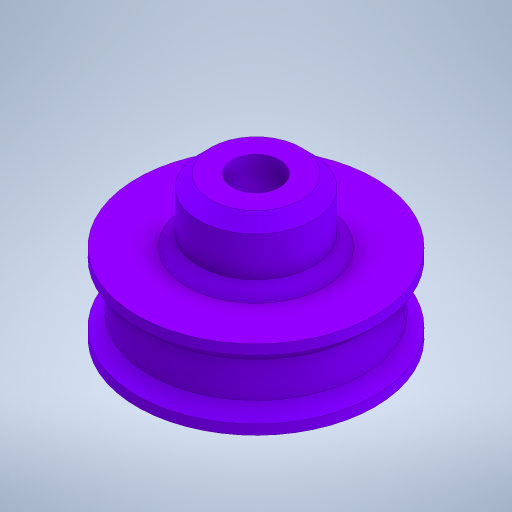
# Autodesk Inventor part: Z Axis Handle
Saved by Autodesk Inventor 2023.1 (Build 271208000, 208)
## iProperties
Created: 2021-10-26
Part Number: Z Axis Handle
Material: Generic
Document SubType Name: Modeling
Designer: xSibe
Density: 1 g/cm^3
Appearance: Plastic Purple
Author: xSibe
Autodesk Inventor part; units mm, degrees
ref_plane "YZ Plane" through (0, 0, 0) normal (1, 0, 0) x (0, 1, 0)
ref_plane "XY Plane" through (0, 0, 0) normal (0, 0, 1) x (1, 0, 0)
sketch "Sketch1" plane through (0, 0, 0) normal (0, 1, 0) x (-1, 0, 0)
  line L0 (1.25, 1.25) -> (-1.25, 1.25)
  line L1 (-1.25, 1.25) -> (-1.25, -1.25)
  line L2 (-1.25, -1.25) -> (1.25, -1.25)
  line L3 (1.25, -1.25) -> (1.25, 1.25)
  line L4 (1.25, 1.25) -> (-1.25, -1.25) construction
  line L5 (-1.25, 1.25) -> (1.25, -1.25) construction
  line L6 (-0.7217, -1.25) -> (-1.4434, 0)
  line L7 (-1.4434, 0) -> (-0.7217, 1.25)
  line L8 (-0.7217, 1.25) -> (0.7217, 1.25)
  line L9 (0.7217, 1.25) -> (1.4434, 0)
  line L10 (1.4434, 0) -> (0.7217, -1.25)
  line L11 (0.7217, -1.25) -> (-0.7217, -1.25)
  line L12 (3.6084, -6.25) -> (7.2169, 0)
  line L13 (7.2169, 0) -> (3.6084, 6.25)
  line L14 (3.6084, 6.25) -> (-3.6084, 6.25)
  line L15 (-3.6084, 6.25) -> (-7.2169, 0)
  line L16 (-7.2169, 0) -> (-3.6084, -6.25)
  line L17 (-3.6084, -6.25) -> (3.6084, -6.25)
  line L18 (3.6084, -6.25) -> (1.2532, -7.1072)
  line L19 (1.2532, -7.1072) -> (-1.2532, -7.1072)
  line L20 (-1.2532, -7.1072) -> (-3.6084, -6.25)
  line L21 (-3.6084, -6.25) -> (-5.5284, -4.6389)
  line L22 (-5.5284, -4.6389) -> (-6.7816, -2.4683)
  line L23 (-6.7816, -2.4683) -> (-7.2169, 0)
  line L24 (-7.2169, 0) -> (-6.7816, 2.4683)
  line L25 (-6.7816, 2.4683) -> (-5.5284, 4.6389)
  line L26 (-5.5284, 4.6389) -> (-3.6084, 6.25)
  line L27 (-3.6084, 6.25) -> (-1.2532, 7.1072)
  line L28 (-1.2532, 7.1072) -> (1.2532, 7.1072)
  line L29 (1.2532, 7.1072) -> (3.6084, 6.25)
  line L30 (3.6084, 6.25) -> (5.5284, 4.6389)
  line L31 (5.5284, 4.6389) -> (6.7816, 2.4683)
  line L32 (6.7816, 2.4683) -> (7.2169, 0)
  line L33 (7.2169, 0) -> (6.7816, -2.4683)
  line L34 (6.7816, -2.4683) -> (5.5284, -4.6389)
  line L35 (5.5284, -4.6389) -> (3.6084, -6.25)
  circle A0 centre (0, 0) radius 3
  line L36 (-0.9887, -5.6072) -> (0.9887, -5.6072)
  line L37 (0.9887, -5.6072) -> (2.8469, -4.9309)
  line L38 (2.8469, -4.9309) -> (4.3617, -3.6599)
  line L39 (4.3617, -3.6599) -> (5.3504, -1.9474)
  line L40 (5.3504, -1.9474) -> (5.6937, 0)
  line L41 (5.6937, 0) -> (5.3504, 1.9474)
  line L42 (5.3504, 1.9474) -> (4.3617, 3.6599)
  line L43 (4.3617, 3.6599) -> (2.8469, 4.9309)
  line L44 (2.8469, 4.9309) -> (0.9887, 5.6072)
  line L45 (0.9887, 5.6072) -> (-0.9887, 5.6072)
  line L46 (-0.9887, 5.6072) -> (-2.8469, 4.9309)
  line L47 (-2.8469, 4.9309) -> (-4.3617, 3.6599)
  line L48 (-4.3617, 3.6599) -> (-5.3504, 1.9474)
  line L49 (-5.3504, 1.9474) -> (-5.6937, 0)
  line L50 (-5.6937, 0) -> (-5.3504, -1.9474)
  line L51 (-5.3504, -1.9474) -> (-4.3617, -3.6599)
  line L52 (-4.3617, -3.6599) -> (-2.8469, -4.9309)
  line L53 (-2.8469, -4.9309) -> (-0.9887, -5.6072)
  circle A1 centre (0, 0) radius 7.2169
  circle A2 centre (0, 0) radius 5.6937
  circle A3 centre (0, 0) radius 15
  circle A4 centre (0, 0) radius 13.5
  point P0 (0, -1.25)
  point P1 (7.2169, 0)
  point P2 (7.2169, 0)
  point P3 (1.2532, 7.1072)
  point P4 (1.2532, 7.1072)
  point P5 (-3.6084, 6.25)
  point P6 (-3.6084, 6.25)
  dimension "d0" = 2.5
  dimension "d1" = 2.5
  dimension "d2" = 5
  dimension "d5" = 6
  dimension "d6" = 1.5
  dimension "d12" = 30
  dimension "d14" = 1.5
  constraints: 108 end point, 6 coincident, 4 midpoint, 3 centre point, 2 parallel, 1 horizontal, 1 horizontal alignment, 1 perpendicular, 77 other
  measures "d0" distance of L2.end L1.end
  measures "d1" distance of L1.end L0.end
  measures "d2" distance between parallel lines of L10 L12
  measures "d5" diameter of A0
  measures "d6" distance between parallel lines of L19 L36
  measures "d12" diameter of A3
  measures "d14" radial gap between concentric circles of A3 A4
ref_plane "Work Plane1" through (0, -4, 0) normal (0, 1, 0) x (-1, 0, 0)
extrude "Extrusion1" add sketch "Sketch1" along normal mid plane 18 contours L17 L16 L15 L14 L13 L12 | L18 L19 L20 L17 | A1 L18 | L12 L33 L34 L35 | L35 A1 | L13 L30 L31 L32 | A1 L33 | L32 A1 | L21 L22 L23 L16 | A1 L21 | L20 A1 | A1 L19 | L34 A1 | L14 L27 L28 L29 | A1 L30 | L29 A1 | L31 A1 | L24 L25 L26 L15 | A1 L24 | L23 A1 | A1 L22 | A1 L27 | L26 A1 | L28 A1 | A1 L25 | L53 L52 L51 L50 L49 L48 L47 L46 L45 L44 L43 L42 L41 L40 L39 L38 L37 L36 | A2 L53 | L36 A2 | L37 A2 | A2 L52 | L38 A2 | A2 L51 | L39 A2 | A2 L50 | L40 A2 | A2 L49 | L41 A2 | A2 L48 | L42 A2 | A2 L47 | L43 A2 | A2 L46 | L44 A2 | A2 L45
extrude "Extrusion2" add sketch "Sketch1" along normal mid plane 10 from surface at -4 contours L17 L16 L15 L14 L13 L12 | L18 L19 L20 L17 | A1 L18 | L12 L33 L34 L35 | L35 A1 | L13 L30 L31 L32 | A1 L33 | L32 A1 | L21 L22 L23 L16 | A1 L21 | L20 A1 | A1 L19 | L34 A1 | L14 L27 L28 L29 | A1 L30 | L29 A1 | L31 A1 | L24 L25 L26 L15 | A1 L24 | L23 A1 | A1 L22 | A1 L27 | L26 A1 | L28 A1 | A1 L25 | A3 | A4
extrude "Extrusion3" cut sketch "Sketch1" along normal mid plane 7.5 from surface at -4 contours A3
chamfer "Chamfer1" distance 1.5 angle 45 4 edges at (13.5, -0.25, 0) (13.5, -7.75, 0) (1.2532, 1, -7.1072) (1.2532, 9, -7.1072)
body "Solid1"
